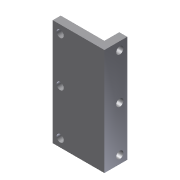
# Autodesk Inventor part: Groin
Saved by Autodesk Inventor 2011 (Build 150239000, 239)
## iProperties
Created: 2010-11-21
Part Number: Groin
Document SubType Name: Modeling
Designer: Milton
Density: 1 g/cm^3
Mass: 2.89707 g
Surface Area: 24.7407 cm^2
Volume: 2.89707 cm^3
Author: Milton
Autodesk Inventor part; units mm, degrees
ref_plane "YZ Plane" through (0, 0, 0) normal (1, 0, 0) x (0, 1, 0)
ref_plane "XZ Plane" through (0, 0, 0) normal (0, 1, 0) x (-1, 0, 0)
ref_plane "XY Plane" through (0, 0, 0) normal (0, 0, 1) x (1, 0, 0)
sketch "Sketch1" plane through (0, 0, 0) normal (0, 0, 1) x (1, 0, 0)
  line L0 (21.4217, 22.24) -> (21.4217, 19.24)
  line L1 (21.4217, 22.24) -> (37.8228, 22.24)
  line L2 (21.4217, 19.24) -> (40.8228, 19.24)
  line L3 (40.8228, 27.84) -> (37.8228, 27.84)
  line L4 (37.8228, 27.84) -> (37.8228, 22.24)
  line L5 (40.8228, 27.84) -> (40.8228, 19.24)
  point P0 (0, 0)
  constraints: 12 end point
extrude "Extrusion1" add sketch "Sketch1" along normal blind 40
sketch "Sketch2" plane through (40.8228, 19.24, 0) normal (1, 0, 0) x (0, 0, -1)
  line L0 (-40, 8.6) -> (-40, 0) projected
  line L1 (0, 8.6) -> (-40, 8.6) projected
  circle A0 centre (-37, 5.8) radius 1.35
  circle A1 centre (-20, 5.8) radius 1.35
  circle A2 centre (-3, 5.8) radius 1.35
  point P0 (0, -19.24)
  dimension "d2" = 2.7
  dimension "d3" = 2.7
  dimension "d4" = 2.8
  dimension "d5" = 2.8
  dimension "d6" = 17
  dimension "d7" = 2.7
  dimension "d8" = 17
  dimension "d9" = 3
  constraints: 3 centre point
  measures "d2" diameter of A0
  measures "d3" diameter of A1
  measures "d4" distance from line of L1 A0.centre
  measures "d5" distance from line of L1 A1.centre
  measures "d6" distance of A1.centre A0.centre
  measures "d7" diameter of A2
  measures "d8" distance of A2.centre A1.centre
  measures "d9" distance from line of L0 A0.centre
extrude "Extrusion2" cut sketch "Sketch2" against normal through all
sketch "Sketch3" plane through (21.4217, 22.24, 0) normal (0, 1, 0) x (1, 0, 0)
  line L0 (16.4011, 0) -> (0, 0) projected
  line L1 (0, 0) -> (0, -40) projected
  circle A0 centre (2.8, -3) radius 1.35
  circle A1 centre (2.8, -20) radius 1.35
  circle A2 centre (2.8, -37) radius 1.35
  point P0 (-21.4217, 0)
  dimension "d12" = 2.7
  dimension "d13" = 3
  dimension "d14" = 2.8
  dimension "d15" = 2.7
  dimension "d16" = 2.7
  dimension "d17" = 17
  dimension "d18" = 17
  constraints: 3 centre point
  measures "d12" diameter of A0
  measures "d13" distance from line of A0.centre L0
  measures "d14" distance from line of L1 A0.centre
  measures "d15" diameter of A1
  measures "d16" diameter of A2
  measures "d17" distance of A2.centre A1.centre
  measures "d18" distance of A1.centre A0.centre
extrude "Extrusion3" cut sketch "Sketch3" against normal through all
body "Solid1"
